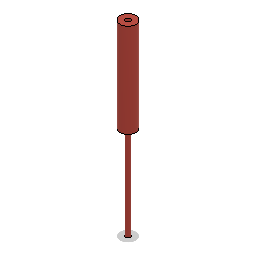
fluke101_2_asm (Autodesk Fusion 360 archive; units mm, degrees)
design "multimeterProbeRed"
Autodesk Fusion 360 part; units mm, degrees
sketch "Sketch1" plane through (0, 0, 0) normal (0, 1, 0) x (1, 0, 0)
  circle A0 centre (0, 0) radius 1.5
  circle A1 centre (0, 0) radius 5
  dimension "d1" = 3
  dimension "d2" = 10
  constraint coincident A0.centre A1.centre
  constraint concentric A0 A1
  measures "d1" diameter of A0
  measures "d2" diameter of A1
extrude "Extrude1" add sketch "Sketch1" along normal blind 60 contours A0 makes body 1
extrude "Extrude2" add sketch "Sketch1" along normal blind 120 and the other way blind -60 separate body makes body 2

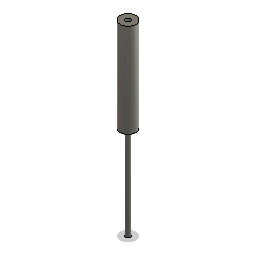
design "multimeterProbe"
Autodesk Fusion 360 part; units mm, degrees
sketch "Sketch1" plane through (0, 0, 0) normal (0, 1, 0) x (1, 0, 0)
  circle A0 centre (0, 0) radius 1.5
  circle A1 centre (0, 0) radius 5
  dimension "d1" = 3
  dimension "d2" = 10
  constraint coincident A0.centre A1.centre
  constraint concentric A0 A1
  measures "d1" diameter of A0
  measures "d2" diameter of A1
extrude "Extrude1" add sketch "Sketch1" along normal blind 60 contours A0 makes body 1
extrude "Extrude2" add sketch "Sketch1" along normal blind 120 and the other way blind -60 separate body makes body 2

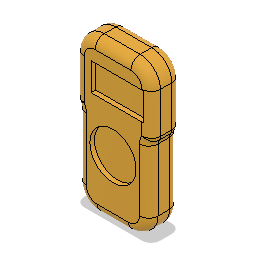
design "fluke101"
Autodesk Fusion 360 part; units mm, degrees
sketch "Sketch1" plane through (0, 0, 0) normal (0, 0, 1) x (1, 0, 0)
  line L0 (31, 65.5) -> (-31, 65.5)
  line L1 (-31, 65.5) -> (-31, -65.5)
  line L2 (-31, -65.5) -> (31, -65.5)
  line L3 (31, -65.5) -> (31, 65.5)
  line L4 (31, 65.5) -> (-31, -65.5) construction
  line L5 (-31, 65.5) -> (31, -65.5) construction
  line L6 (-31, 65.5) -> (-33, 65.5)
  line L7 (-33, 65.5) -> (-33, 10.5)
  line L8 (-33, 10.5) -> (-31, 10.5)
  line L9 (31, 10.5) -> (33, 10.5)
  line L10 (33, 10.5) -> (33, 65.5)
  line L11 (33, 65.5) -> (31, 65.5)
  line L12 (26, 47.5) -> (-19, 47.5)
  line L13 (-19, 47.5) -> (-19, 23.5)
  line L14 (-19, 23.5) -> (26, 23.5)
  line L15 (26, 23.5) -> (26, 47.5)
  line L16 (26, 47.5) -> (-19, 23.5) construction
  line L17 (-19, 47.5) -> (26, 23.5) construction
  circle A0 centre (0, -14.5) radius 20
  point P0 (3.5, 35.5)
  dimension "d1" = 62
  dimension "d2" = 131
  dimension "d3" = 2
  dimension "d4" = 2
  dimension "d6" = 76
  dimension "d7" = 76
  dimension "d16" = 45
  dimension "d17" = 24
  dimension "d18" = 18
  dimension "d19" = 40
  dimension "d20" = 80
  constraint horizontal L0
  constraint perpendicular L0 L1
  constraint parallel L0 L2
  constraint parallel L1 L3
  constraint coincident L4 origin
  constraint coincident L5 origin
  constraint perpendicular L1 L6
  constraint perpendicular L6 L7
  constraint coincident L1 L8.end
  constraint perpendicular L1 L8
  constraint coincident L3 L9.start
  constraint perpendicular L3 L9
  constraint perpendicular L0 L10
  constraint perpendicular L3 L11
  constraint horizontal L12
  constraint perpendicular L12 L13
  constraint parallel L12 L14
  constraint parallel L13 L15
  constraint coincident L16 P0
  constraint coincident L17 P0
  measures "d1" distance of L1.end L2.end
  measures "d2" distance of L0.end L1.end
  measures "d3" distance of L1 L7
  measures "d4" distance of L3 L10
  measures "d6" vertical distance of L1.end L7.end
  measures "d7" vertical distance of L2.end L9.end
  measures "d16" distance of L13.end L14.end
  measures "d17" distance of L12.end L13.end
  measures "d18" distance of L0 L12
  measures "d19" diameter of A0
  measures "d20" distance of L0 A0.centre
extrude "Extrude1" add sketch "Sketch1" against normal blind 26 contours L0 L1 L2 L3 | L3 L9 L10 L11 | L1 L6 L7 L8 | L12 L13 L14 L15 | A0
fillet "Fillet1" radius 6 4 edges at (31, 10.5, -13) (-31, 10.5, -13) (-33, 10.5, -13) (33, 10.5, -13)
fillet "Fillet2" radius 8 20 edges at (0, 65.5, 0) (-33, 39.0806, 0) (-32.7446, 10.9291, 0) (-31.2554, 7.7599, 0) (-31, -29.7361, 0) (31, -29.7361, 0) (31.2554, 7.7599, 0) (32.7446, 10.9291, 0) (33, 39.0806, 0) (0, -65.5, 0) (0, -65.5, -26) (33, 39.0806, -26) (32.7446, 10.9291, -26) (31.2554, 7.7599, -26) (31, -29.7361, -26) (-31, -29.7361, -26) (-31.2554, 7.7599, -26) (-32.7446, 10.9291, -26) (-33, 39.0806, -26) (0, 65.5, -26)
fillet "Fillet3" radius 17.5 12 edges at (30.6569, 63.1569, -2.3431) (33, 65.5, -13) (30.6569, 63.1569, -23.6569) (-30.6569, 63.1569, -23.6569) (-33, 65.5, -13) (-30.6569, 63.1569, -2.3431) (-28.6569, -63.1569, -2.3431) (-31, -65.5, -13) (-28.6569, -63.1569, -23.6569) (28.6569, -63.1569, -2.3431) (31, -65.5, -13) (28.6569, -63.1569, -23.6569)
extrude "Extrude2" cut sketch "Sketch1" against normal blind 4 contours L12 L13 L14 L15 | A0
